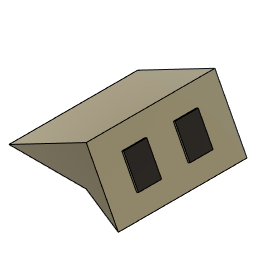
hautaileron v6 (Autodesk Fusion 360 design; units mm, degrees)
Autodesk Fusion 360 part; units mm, degrees
sketch "Esquisse1" plane through (0, 0, 0) normal (0, 1, 0) x (1, 0, 0)
  line L0 (0, 0) -> (60, 0)
  line L1 (60, 0) -> (84.9586, 16.6453)
  line L2 (84.9586, 16.6453) -> (60.0163, -31.2683)
  line L3 (60.0163, -31.2683) -> (0, 0)
  line L4 (61.2115, -4) -> (74.217, 4.6736)
  line L5 (74.217, 4.6736) -> (58.3159, -25.8721)
  line L6 (58.3159, -25.8721) -> (16.3347, -4)
  line L7 (16.3347, -4) -> (61.2115, -4)
  dimension "d1" = 60
  dimension "d2" = 30
  dimension "d3" = 146.3
  dimension "d4" = 28.8
  dimension "d5" = 54.017
  dimension "d6" = 4
  constraint coincident L0.start L3.end
  constraint horizontal L0
  measures "d1" distance of L0.start L0.end
  measures "d2" distance of L0.end L1.end
  measures "d3" angle of L0 L1
  measures "d4" angle of L1 L2
  measures "d5" distance of L1.end L2.end
extrude "Extrusion1" add sketch "Esquisse1" along normal blind 100
sketch "Esquisse2" plane through (0, 0, 0) normal (0, 1, 0) x (1, 0, 0)
  line L0 (0, 0) -> (60, 0)
  line L1 (60, 0) -> (84.9586, 16.6453)
  line L2 (84.9586, 16.6453) -> (60, -31.2598)
  line L3 (60, -31.2598) -> (0, 0)
  dimension "d9" = 60
  dimension "d10" = 146.3
  dimension "d11" = 30
  dimension "d12" = 54.017
  dimension "d13" = 28.78
  constraint coincident L0.start L3.end
  constraint horizontal L0
  measures "d9" distance of L0.start L0.end
  measures "d10" angle of L0 L1
  measures "d11" distance of L0.end L1.end
  measures "d12" distance of L1.end L2.end
  measures "d13" angle of L1 L2
sketch "Esquisse3" plane through (0, 0, 0) normal (0, 1, 0) x (1, 0, 0)
extrude "Extrusion2" add sketch "Esquisse2" along normal blind 4
sketch "Esquisse5" plane through (0, 100, 0) normal (0, 1, 0) x (-1, 0, 0)
  line L0 (-58.3159, 25.8721) -> (-16.3347, 4)
  line L1 (-16.3347, 4) -> (-61.2115, 4)
  line L2 (-61.2115, 4) -> (-74.217, -4.6736)
  line L3 (-74.217, -4.6736) -> (-58.3159, 25.8721)
  line L4 (-60.0163, 31.2683) -> (-84.9586, -16.6453)
  line L5 (-84.9586, -16.6453) -> (-60, 0)
  line L6 (-60, 0) -> (0, 0)
  line L7 (0, 0) -> (-60.0163, 31.2683)
sketch "Esquisse6" plane through (0, 100, 0) normal (0, 1, 0) x (-1, 0, 0)
  line L0 (0, 0) -> (-60, 0)
  line L1 (-60, 0) -> (-84.9586, -16.6453)
  line L2 (-84.9586, -16.6453) -> (-60.0133, 31.2668)
  line L3 (-60.0133, 31.2668) -> (0, 0)
  dimension "d21" = 60
  dimension "d22" = 146.3
  dimension "d23" = 30
  dimension "d24" = 54.017
  dimension "d25" = 28.796
  constraint coincident L0.start L3.end
  constraint horizontal L0
  measures "d21" distance of L0.start L0.end
  measures "d22" angle of L0 L1
  measures "d23" distance of L0.end L1.end
  measures "d24" distance of L1.end L2.end
  measures "d25" angle of L1 L2
extrude "Extrusion3" add sketch "Esquisse6" against normal blind 4
sketch "Esquisse7" plane through (60.0269, 0, 31.248) normal (0.887011, 0, 0.461749) x (0, 1, 0)
  line L0 (0, 0.0229) -> (0, -53.9941)
  line L1 (0, -53.9941) -> (100, -53.9941)
  line L2 (100, -53.9941) -> (100, 0.0229)
  line L3 (100, 0.0229) -> (0, 0.0229)
  line L4 (39, -39.4856) -> (21, -39.4856)
  line L5 (21, -39.4856) -> (21, -14.4856)
  line L6 (21, -14.4856) -> (39, -14.4856)
  line L7 (39, -14.4856) -> (39, -39.4856)
  line L8 (39, -39.4856) -> (21, -14.4856) construction
  line L9 (21, -39.4856) -> (39, -14.4856) construction
  line L10 (61, -39.4856) -> (79, -39.4856)
  line L11 (79, -39.4856) -> (79, -14.4856)
  line L12 (79, -14.4856) -> (61, -14.4856)
  line L13 (61, -14.4856) -> (61, -39.4856)
  line L14 (61, -39.4856) -> (79, -14.4856) construction
  line L15 (79, -39.4856) -> (61, -14.4856) construction
  point P0 (30, -26.9856)
  point P1 (70, -26.9856)
  dimension "d32" = 18
  dimension "d33" = 25
  dimension "d34" = 18
  dimension "d35" = 25
  constraint horizontal L4
  constraint perpendicular L4 L5
  constraint parallel L4 L6
  constraint parallel L5 L7
  constraint coincident L8 P0
  constraint coincident L9 P0
  constraint horizontal L10
  constraint perpendicular L10 L11
  constraint parallel L10 L12
  constraint parallel L11 L13
  constraint coincident L14 P1
  constraint coincident L15 P1
  measures "d32" distance of L5.end L6.end
  measures "d33" distance of L4.end L5.end
  measures "d34" distance of L11.end L12.end
  measures "d35" distance of L10.end L11.end
extrude "Extrusion4" add sketch "Esquisse7" along normal blind 1.5 contours L4 L5 L6 L7 | L10 L11 L12 L13
